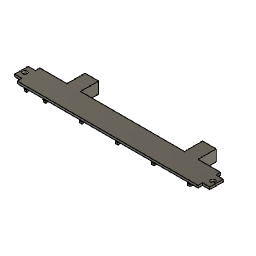
led strip bar v2 (Autodesk Fusion 360 design; units mm, degrees)
Autodesk Fusion 360 part; units mm, degrees
sketch "Sketch1" plane through (0, 0, 0) normal (0, 0, 1) x (1, 0, 0)
  line L0 (100, -12.5) -> (-100, -12.5)
  line L1 (-100, -12.5) -> (-100, 12.5)
  line L2 (-100, 12.5) -> (100, 12.5)
  line L3 (100, 12.5) -> (100, -12.5)
  line L4 (100, -12.5) -> (-100, 12.5) construction
  line L5 (-100, -12.5) -> (100, 12.5) construction
  line L6 (-100, 12.5) -> (-70, 12.5) construction
  line L7 (-70, 12.5) -> (-70, 10.5) construction
  line L8 (-70, 10.5) -> (-100, 10.5) construction
  line L9 (-100, 10.5) -> (-100, 12.5) construction
  line L10 (100, 12.5) -> (70, 12.5) construction
  line L11 (70, 12.5) -> (70, 10.5) construction
  line L12 (70, 10.5) -> (100, 10.5) construction
  line L13 (100, 10.5) -> (100, 12.5) construction
  line L14 (-70, 12.5) -> (-55, 12.5)
  line L15 (-55, 12.5) -> (-55, 32.5)
  line L16 (-55, 32.5) -> (-70, 32.5)
  line L17 (-70, 32.5) -> (-70, 12.5)
  line L18 (60, 32.5) -> (60, 12.5)
  line L19 (75, 12.5) -> (75, 32.5)
  line L20 (75, 32.5) -> (60, 32.5)
  line L21 (100, -7.5328) -> (108, -7.5328)
  line L22 (108, -7.5328) -> (108, 7.4672)
  line L23 (108, 7.4672) -> (100, 7.4672)
  line L24 (100, 7.4672) -> (100, -7.5328)
  circle A0 centre (104, 0) radius 2.5
  line L25 (-108, 7.604) -> (-108, -7.396)
  circle A1 centre (-104, 0) radius 2.5
  line L26 (-100, 7.604) -> (-108, 7.604)
  line L27 (-108, -7.396) -> (-100, -7.396)
  line L28 (60, 12.5) -> (75, 12.5)
  dimension "d1" = 200
  dimension "d2" = 25
  dimension "d3" = 30
  dimension "d4" = 2
  dimension "d5" = 30
  dimension "d6" = 2
  dimension "d7" = 15
  dimension "d8" = 20
  dimension "d9" = 15
  dimension "d10" = 20
  dimension "d11" = 15
  dimension "d12" = 8
  dimension "d13" = 5
  dimension "d14" = 15
  dimension "d15" = 8
  dimension "d16" = 5
  constraint horizontal L0
  constraint perpendicular L0 L1
  constraint parallel L0 L2
  constraint parallel L1 L3
  constraint coincident L4 origin
  constraint coincident L5 origin
  constraint horizontal L6
  constraint vertical L7
  constraint horizontal L8
  constraint vertical L9
  constraint horizontal L10
  constraint vertical L11
  constraint horizontal L12
  constraint vertical L13
  constraint horizontal L14
  constraint vertical L15
  constraint horizontal L16
  constraint vertical L17
  constraint vertical L19
  constraint horizontal L20
  constraint vertical L18
  constraint horizontal L21
  constraint vertical L22
  constraint horizontal L23
  constraint vertical L24
  constraint coincident L3 L21.start
  constraint perpendicular L19 L28
  measures "d1" distance of L1.end L2.end
  measures "d2" distance of L0.end L1.end
  measures "d3" distance of L1.end L6.end
  measures "d4" distance of L1.end L8.end
  measures "d5" distance of L2.end L10.end
  measures "d6" distance of L2.end L12.end
  measures "d7" distance of L6.end L14.end
  measures "d8" distance of L6.end L16.end
  measures "d9" distance of L19.start L18.end
  measures "d10" distance of L18.start L18.end
  measures "d11" distance of L21.start L23.end
  measures "d12" distance of L21.start L21.end
  measures "d13" diameter of A0
  measures "d14" distance of L27.end L26.start
  measures "d15" distance of L25.start L26.start
  measures "d16" diameter of A1
extrude "Extrude1" add sketch "Sketch1" along normal blind 2.5
extrude "Extrude2" add sketch "Sketch1" against normal blind 7.5 contours L2 L18 L19 L20 L28 | L2 L14 L15 L16 L17
sketch "Sketch2" plane through (0, 0, 0) normal (0, 0, 1) x (1, 0, 0)
  line L0 (-55, 12.5) -> (-65, 12.5)
  line L1 (-65, 12.5) -> (-65, 10)
  line L2 (-65, 10) -> (-55, 10)
  line L3 (-55, 10) -> (-55, 12.5)
  line L4 (70, 12.5) -> (60, 12.5)
  line L5 (60, 12.5) -> (60, 10)
  line L6 (60, 10) -> (70, 10)
  line L7 (70, 10) -> (70, 12.5)
  point P0 (-55, 12.5)
  point P1 (70, 12.5)
  constraint horizontal L0
  constraint vertical L1
  constraint horizontal L2
  constraint vertical L3
  constraint coincident P0 L0.start
  constraint horizontal L4
  constraint vertical L5
  constraint horizontal L6
  constraint vertical L7
  constraint coincident P1 L4.start
extrude "Extrude3" add sketch "Sketch2" against normal blind 7.5
chamfer "Chamfer1" distance 5 angle 45 2 edges at (65, 10, -7.5) (-60, 10, -7.5)
sketch "Sketch3" plane through (0, 32.5, 0) normal (0, 1, 0) x (-1, 0, 0)
  line L0 (70, -7.5) -> (70, 2.5)
  line L1 (70, 2.5) -> (55, 2.5)
  line L2 (55, 2.5) -> (55, -7.5)
  line L3 (55, -7.5) -> (70, -7.5)
  circle A0 centre (63.0103, -3.6529) radius 2.5
  circle A1 centre (-67.513, -3.4918) radius 2.5
  dimension "d24" = 5
  dimension "d25" = 5
  measures "d24" diameter of A0
  measures "d25" diameter of A1
extrude "Extrude4" cut sketch "Sketch3" against normal blind 15 contours A0 | A1
ref_plane "WorkPlane1" through (-62.5, 20, -2.5) normal (0, 1, 0) x (-1, 0, 0)
sketch "Sketch4" plane through (-65, 20, -4.8909) normal (0, 1, 0) x (1, 0, 0)
  circle A0 centre (2, -1.2336) radius 4.3
  circle A1 centre (132.5, -1.4) radius 4.3
  dimension "d31" = 8.6
  dimension "d32" = 8.6
  measures "d31" diameter of A0
  measures "d32" diameter of A1
extrude "Extrude5" add 2 faces at (-65, 26.6667, -7.5) (65, 26.6667, -7.5) along direction (0, 0, -1) blind 2.5
extrude "Extrude6" cut sketch "Sketch4" along normal blind 8
sketch "Sketch5" plane through (0, 0, 0) normal (0, 0, 1) x (1, 0, 0)
  line L0 (95, -6.5) -> (95, 6.5) construction
  line L1 (-95, 6.5) -> (-95, -6.5) construction
  line L2 (-95, -6.5) -> (95, 6.5) construction
  line L3 (95, -6.5) -> (-95, 6.5) construction
  line L4 (87.4552, 6.5) -> (84.4552, 6.5)
  line L5 (84.4552, 6.5) -> (84.4552, 9)
  line L6 (84.4552, 9) -> (87.4552, 9)
  line L7 (87.4552, 9) -> (87.4552, 6.5)
  line L8 (87.4552, 6.5) -> (84.4552, 6.5) construction
  line L9 (84.4552, 6.5) -> (84.4552, -6.5258) construction
  line L10 (84.4552, -6.5258) -> (87.4552, -6.5258) construction
  line L11 (87.4552, -6.5258) -> (87.4552, 6.5) construction
  line L12 (87.4552, -6.5258) -> (84.4552, -6.5258)
  line L13 (84.4552, -6.5258) -> (84.4552, -8.5258)
  line L14 (84.4552, -8.5258) -> (87.4552, -8.5258)
  line L15 (87.4552, -8.5258) -> (87.4552, -6.5258)
  line L16 (44.4552, 6.5) -> (44.4552, 9)
  line L17 (44.4552, -6.5258) -> (47.4552, -6.5258) construction
  line L18 (44.4552, -6.5258) -> (47.4552, -6.5258) construction
  line L19 (44.4552, -6.5258) -> (44.4552, -8.5258)
  line L20 (44.4552, -8.5258) -> (47.4552, -8.5258)
  line L21 (47.4552, -8.5258) -> (47.4552, -6.5258)
  line L22 (47.4552, 6.5) -> (44.4552, 6.5) construction
  line L23 (44.4552, 6.5) -> (44.4552, 9)
  line L24 (44.4552, 9) -> (47.4552, 9)
  line L25 (47.4552, 9) -> (47.4552, 6.5)
  line L26 (4.4552, 6.5) -> (4.4552, 9)
  line L27 (7.4552, 9) -> (7.4552, 6.5)
  line L28 (4.4552, 9) -> (7.4552, 9)
  line L29 (7.4552, -8.5258) -> (7.4552, -6.5258)
  line L30 (4.4552, -8.5258) -> (7.4552, -8.5258)
  line L31 (4.4552, -6.5258) -> (4.4552, -8.5258)
  line L32 (-75.5448, 9) -> (-72.5448, 9)
  line L33 (-75.5448, 6.5) -> (-75.5448, 9)
  line L34 (-72.5448, 9) -> (-72.5448, 6.5)
  line L35 (-75.5448, -8.5258) -> (-72.5448, -8.5258)
  line L36 (-72.5448, -8.5258) -> (-72.5448, -6.5258)
  line L37 (-75.5448, -6.5258) -> (-75.5448, -8.5258)
  line L38 (-35.5448, -6.5258) -> (-35.5448, -8.5258)
  line L39 (-35.5448, -8.5258) -> (-32.5448, -8.5258)
  line L40 (-32.5448, -8.5258) -> (-32.5448, -6.5258)
  line L41 (-35.5448, 6.5) -> (-35.5448, 9)
  line L42 (-35.5448, 9) -> (-32.5448, 9)
  line L43 (-32.5448, 9) -> (-32.5448, 6.5)
  line L44 (-96.5448, 6.5) -> (-96.5448, 9)
  line L45 (-93.5448, 9) -> (-93.5448, 6.5)
  line L46 (-96.5448, 9) -> (-93.5448, 9)
  line L47 (-96.5448, -6.5258) -> (-96.5448, -8.5258)
  line L48 (-96.5448, -8.5258) -> (-93.5448, -8.5258)
  line L49 (-93.5448, -8.5258) -> (-93.5448, -6.5258)
  line L50 (-96.5448, -6.5258) -> (-93.5448, -6.5258)
  line L51 (-96.5448, 6.5) -> (-93.5448, 6.5)
  line L52 (-75.5448, 6.5) -> (-72.5448, 6.5)
  line L53 (-75.5448, -6.5258) -> (-75, -6.5258)
  line L54 (-75, -6.5258) -> (-72.5448, -6.5258)
  line L55 (-35.5448, 6.5) -> (-32.5448, 6.5)
  line L56 (-35.5448, -6.5258) -> (-32.5448, -6.5258)
  line L57 (4.4552, -6.5258) -> (7.4552, -6.5258)
  line L58 (4.4552, 6.5) -> (7.4552, 6.5)
  line L59 (44.4552, -6.5258) -> (47.4552, -6.5258)
  line L60 (44.4552, 6.5) -> (47.4552, 6.5)
  dimension "d37" = 190
  dimension "d38" = 13
  dimension "d39" = 3
  dimension "d40" = 2.5
  dimension "d41" = 3
  dimension "d42" = 3
  dimension "d43" = 2
  dimension "d52" = 3
  dimension "d53" = 2.5
  dimension "d54" = 3
  dimension "d55" = 3
  dimension "d56" = 2
  dimension "d57" = 2.5
  dimension "d58" = 3
  dimension "d59" = 2
  dimension "d60" = 2.5
  dimension "d61" = 3
  dimension "d62" = 2
  dimension "d63" = 2.5
  dimension "d64" = 3
  dimension "d65" = 2
  dimension "d66" = 2.5
  dimension "d67" = 3
  dimension "d68" = 2
  constraint parallel L0 L1
  constraint coincident L2 origin
  constraint coincident L3 origin
  constraint horizontal L4
  constraint vertical L5
  constraint horizontal L6
  constraint vertical L7
  constraint horizontal L8
  constraint vertical L9
  constraint horizontal L10
  constraint vertical L11
  constraint horizontal L12
  constraint vertical L13
  constraint horizontal L14
  constraint vertical L15
  constraint vertical L16
  constraint horizontal L17
  constraint vertical L23
  constraint horizontal L24
  constraint vertical L25
  constraint horizontal L22
  constraint horizontal L18
  constraint vertical L19
  constraint horizontal L20
  constraint vertical L21
  constraint vertical L26
  constraint horizontal L28
  constraint vertical L27
  constraint vertical L31
  constraint horizontal L30
  constraint vertical L29
  constraint vertical L41
  constraint horizontal L42
  constraint vertical L43
  constraint vertical L38
  constraint horizontal L39
  constraint vertical L40
  constraint vertical L33
  constraint horizontal L32
  constraint vertical L34
  constraint vertical L37
  constraint horizontal L35
  constraint vertical L36
  constraint vertical L44
  constraint horizontal L46
  constraint vertical L45
  constraint vertical L47
  constraint horizontal L48
  constraint vertical L49
  constraint perpendicular L49 L50
  constraint perpendicular L45 L51
  constraint perpendicular L34 L52
  constraint perpendicular L37 L53
  constraint perpendicular L36 L54
  constraint perpendicular L43 L55
  constraint perpendicular L40 L56
  constraint perpendicular L29 L57
  constraint perpendicular L27 L58
  constraint perpendicular L19 L59
  measures "d37" distance of L0.end L1.start
  measures "d38" distance of L0.start L0.end
  measures "d39" distance of L4.start L4.end
  measures "d40" distance of L4.start L6.end
  measures "d41" distance of L4.start L4.end
  measures "d42" distance of L10.end L9.end
  measures "d43" distance of L10.end L14.end
  measures "d52" distance of L16.start L22.start
  measures "d53" distance of L22.start L24.end
  measures "d54" distance of L16.start L22.start
  measures "d55" distance of L17.start L17.end
  measures "d56" distance of L20.end L17.end
  measures "d57" distance of L27.end L27.start
  measures "d58" distance of L31.start L29.end
  measures "d59" distance of L29.start L29.end
  measures "d60" distance of L43.end L42.end
  measures "d61" distance of L38.start L40.end
  measures "d62" distance of L39.end L40.end
  measures "d63" distance of L34.end L32.end
  measures "d64" distance of L36.end L37.start
  measures "d65" distance of L36.end L35.end
  measures "d66" distance of L45.start L45.end
  measures "d67" distance of L47.start L49.end
  measures "d68" distance of L49.end L48.end
extrude "Extrude7" add sketch "Sketch5" against normal blind 5 contours L4 L5 L6 L7 | L12 L13 L14 L15
extrude "Extrude9" add sketch "Sketch5" against normal blind 5 contours L16 L23 L24 L25 L60 | L19 L20 L21 L59 | L26 L27 L28 L58 | L29 L30 L31 L57 | L32 L33 L34 L52 | L35 L36 L37 L53 L54 | L38 L39 L40 L56 | L41 L42 L43 L55 | L44 L45 L46 L51 | L47 L48 L49 L50
sketch "Sketch7" plane through (0, 0, -5) normal (0, 0, -1) x (1, 0, 0)
  line L0 (84.4552, -9) -> (87.4552, -9)
  line L1 (87.4552, -9) -> (87.4552, -6.5)
  line L2 (87.4552, -6.5) -> (84.4552, -6.5)
  line L3 (84.4552, -6.5) -> (84.4552, -9)
  line L4 (87.4552, -9) -> (84.4598, -9)
  line L5 (84.4598, -9) -> (84.4598, 8.5262)
  line L6 (84.4598, 8.5262) -> (87.4552, 8.5262)
  line L7 (87.4552, 8.5262) -> (87.4552, -9)
  line L8 (47.4598, -8.9738) -> (44.4598, -8.9738)
  line L9 (44.4598, -8.9738) -> (44.4598, 8.5262)
  line L10 (44.4598, 8.5262) -> (47.4598, 8.5262)
  line L11 (47.4598, 8.5262) -> (47.4598, -8.9738)
  line L12 (7.4598, -8.9738) -> (4.4598, -8.9738)
  line L13 (4.4598, -8.9738) -> (4.4598, 8.5262)
  line L14 (4.4598, 8.5262) -> (7.4598, 8.5262)
  line L15 (7.4598, 8.5262) -> (7.4598, -8.9738)
  line L16 (-32.5, -9) -> (-35.5, -9)
  line L17 (-35.5, -9) -> (-35.5, 8.5)
  line L18 (-35.5, 8.5) -> (-32.5, 8.5)
  line L19 (-32.5, 8.5) -> (-32.5, -9)
  line L20 (-72.5, -9) -> (-75.5, -9)
  line L21 (-75.5, -9) -> (-75.5, 8.5)
  line L22 (-75.5, 8.5) -> (-72.5, 8.5)
  line L23 (-72.5, 8.5) -> (-72.5, -9)
  line L24 (-93.5, -9) -> (-96.5, -9)
  line L25 (-96.5, -9) -> (-96.5, 8.5)
  line L26 (-96.5, 8.5) -> (-93.5, 8.5)
  line L27 (-93.5, 8.5) -> (-93.5, -9)
  dimension "d71" = 3
  dimension "d72" = 17.5
  dimension "d73" = 3
  dimension "d74" = 17.5
  dimension "d75" = 3
  dimension "d76" = 17.5
  dimension "d77" = 3
  dimension "d78" = 17.5
  constraint horizontal L4
  constraint vertical L5
  constraint horizontal L6
  constraint vertical L7
  constraint coincident L0.end L1.start
  constraint horizontal L8
  constraint vertical L9
  constraint horizontal L10
  constraint vertical L11
  constraint horizontal L12
  constraint vertical L13
  constraint horizontal L14
  constraint vertical L15
  constraint horizontal L16
  constraint vertical L17
  constraint horizontal L18
  constraint vertical L19
  constraint horizontal L20
  constraint vertical L21
  constraint horizontal L22
  constraint vertical L23
  constraint horizontal L24
  constraint vertical L25
  constraint horizontal L26
  constraint vertical L27
  measures "d71" distance of L12.start L12.end
  measures "d72" distance of L12.start L14.end
  measures "d73" distance of L16.start L16.end
  measures "d74" distance of L16.start L18.end
  measures "d75" distance of L20.start L20.end
  measures "d76" distance of L20.start L22.end
  measures "d77" distance of L24.start L24.end
  measures "d78" distance of L24.start L26.end
extrude "Extrude10" add sketch "Sketch7" along normal blind 2 contours L0 L1 L2 L4 L5 L7 | L2 L5 L6 L7 | L8 L9 L10 L11 | L12 L13 L14 L15 | L16 L17 L18 L19 | L20 L21 L22 L23 | L24 L25 L26 L27
sketch "Sketch8" plane through (0, 0, 0) normal (0, 0, 1) x (1, 0, 0)
  line L0 (95, 6.5) -> (-100, 6.5)
  line L1 (-100, 6.5) -> (-100, -6.5258)
  line L2 (-100, -6.5258) -> (95, -6.5258)
  line L3 (95, -6.5258) -> (95, 6.5)
  line L4 (-100, -12.5) -> (-100, 12.5)
  line L5 (95, 6.5) -> (100, 6.5)
  line L6 (100, 6.5) -> (100, -6.5)
  line L7 (100, -6.5) -> (95, -6.5)
  line L8 (95, -6.5) -> (95, 6.5)
  point P0 (95, 6.5)
  dimension "d81" = 13
  constraint horizontal L0
  constraint vertical L1
  constraint horizontal L2
  constraint vertical L3
  constraint coincident L1.end L4
  constraint coincident P0 L0.start
  constraint horizontal L5
  constraint vertical L6
  constraint horizontal L7
  constraint vertical L8
  measures "d81" distance of P0 L7.end
extrude "Extrude11" cut sketch "Sketch8" along normal blind 1
extrude "Extrude12" add 1 faces at (70, 11.6667, -2.5) along direction (1, 0, 0) blind 5
extrude "Extrude13" add 1 faces at (-65, 11.6667, -2.5) along direction (-1, 0, 0) blind 5
extrude "Extrude14" cut sketch "Sketch4" against normal blind 17
